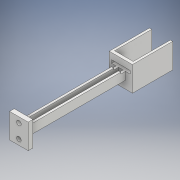
# Autodesk Inventor part: learnbotAgarreServo
Saved by Autodesk Inventor 2017 (Build 210142000, 142)
## iProperties
Part Number: learnbotAgarreServo
Material: Genérico
Document SubType Name: Modeling
Designer: rober
Density: 1 g/cm^3
Appearance: Valor por defecto
Author: rober
Autodesk Inventor part; units mm, degrees
ref_plane "YZ Plane" through (0, 0, 0) normal (1, 0, 0) x (0, 1, 0)
ref_plane "XZ Plane" through (0, 0, 0) normal (0, 1, 0) x (-1, 0, 0)
ref_plane "XY Plane" through (0, 0, 0) normal (0, 0, 1) x (1, 0, 0)
sketch "Boceto1" plane through (0, 0, 0) normal (0, 0, 1) x (1, 0, 0)
  line L0 (-0.3, 9.187) -> (-0.3, 6.787)
  line L1 (-0.3, 6.787) -> (0.9, 6.787)
  line L2 (0.9, 6.787) -> (0.9, 9.187)
  line L3 (0.9, 9.187) -> (1.05, 9.187)
  line L4 (1.05, 9.187) -> (1.05, 6.587)
  line L5 (0, 6.587) -> (-0.45, 6.587)
  line L6 (-0.45, 6.587) -> (-0.45, 9.187)
  line L7 (-0.45, 9.187) -> (-0.3, 9.187)
  line L8 (0.6, 0) -> (0.6, 6.587)
  line L9 (0.45, 6.587) -> (0.15, 6.587)
  line L10 (0, 6.587) -> (0, 0)
  line L11 (0, 0.3) -> (0.6, 0.3)
  line L12 (0.15, 0.3) -> (0.15, 6.587)
  line L13 (0.45, 0.3) -> (0.45, 6.587)
  line L14 (0.6, 6.587) -> (1.05, 6.587)
  line L15 (0, 0) -> (0.6, 0)
  point P0 (0, 0)
  constraints: 32 end point, 4 point on line
extrude "Extrusión1" add sketch "Boceto1" along normal blind 1.6 contours L0 L1 L2 L3 L4 L14 L8 L11 L13 L9 L12 L10 L5 L6 L7 | L11 L8 L15 L10
sketch "Boceto2" plane through (-0.3, 6.787, 0) normal (0, 1, 0) x (1, 0, 0)
  line L0 (1.2, 0) -> (0, 0) projected
  line L1 (0, 0) -> (0, -1.6) projected
  line L2 (1.2, -1.6) -> (0, -1.6) projected
  line L3 (1.2, 0) -> (1.2, -1.6) projected
  line L4 (0, -1.6) -> (0, -1.2)
  line L5 (0, -1.2) -> (0, -1)
  line L6 (0, -1) -> (1.2, -1)
  line L7 (1.2, 0) -> (1.2, -1.6) projected
  line L8 (0, -1.2) -> (1.2, -1.2)
  line L9 (1.2, -1.2) -> (1.2, -1)
  point P0 (0.3, 0)
  dimension "d2" = 0.4
  dimension "d3" = 0.2
  dimension "d4" = 1.2
  constraints: 10 end point, 4 point on line, 1 perpendicular
  measures "d2" distance of L1.end L4.end
  measures "d3" distance of L4.end L5.end
  measures "d4" distance of L4.end L8.end
extrude "Extrusión2" cut sketch "Boceto2" against normal blind 0.5 contours L3 L8 L1 L6
sketch "Boceto3" plane through (0.6, 0, 0) normal (1, 0, 0) x (0, 0, -1)
  line L0 (-1.6, 0.3) -> (0, 0.3) projected
  line L1 (-1, 6.587) -> (-1, 6.287) projected
  line L2 (-1, 6.287) -> (-1.2, 6.287) projected
  line L3 (-1.2, 6.287) -> (-1.2, 6.587) projected
  line L4 (-1.2, 6.587) -> (-1.6, 6.587) projected
  line L5 (-1.6, 0) -> (-1.6, 6.587) projected
  line L6 (0, 0) -> (-1.6, 0) projected
  line L7 (0, 0) -> (0, 6.587) projected
  line L8 (0, 6.587) -> (-1, 6.587) projected
  line L9 (-1.6, 0.3) -> (-1.6, 6.587) projected
  line L10 (-1.6, 0.3) -> (-1.2, 0.3)
  line L11 (-1.2, 0.3) -> (-1.2, 6.587)
  line L12 (-1.6, 6.587) -> (-1.2, 6.587)
  line L13 (-1.2, 6.587) -> (-1.2, 0.3)
  line L14 (-1.2, 0.3) -> (-1.6, 0.3)
  line L15 (-1.6, 0.3) -> (-1.6, 6.587)
  line L16 (0, 0.3) -> (0, 6.587) projected
  line L17 (0, 0.3) -> (-0.4, 0.3)
  line L18 (0, 0.3) -> (-1.6, 0.3) projected
  line L19 (0, 6.587) -> (-1.6, 6.587) projected
  line L20 (0, 6.587) -> (-0.4, 6.587)
  line L21 (-0.4, 6.587) -> (-0.4, 0.3)
  line L22 (-0.4, 0.3) -> (0, 0.3)
  line L23 (0, 0.3) -> (0, 6.587)
  point P0 (0, 0)
  dimension "d7" = 0.4
  dimension "d8" = 0.4
  constraints: 22 end point, 4 parallel, 2 horizontal, 2 perpendicular, 2 point on line
  measures "d7" distance of L0.start L10.end
  measures "d8" distance of L0.end L17.end
extrude "Extrusión3" cut sketch "Boceto3" against normal blind 0.9 contours L5 L4 L3 L11 L0 | L21 L8 L7 L0
sketch "Boceto4" plane through (0, 0.3, 0) normal (0, 1, 0) x (1, 0, 0)
  line L0 (0, 0) -> (0.6, 0) projected
  line L1 (0.6, 0) -> (0.6, -1.6) projected
  line L2 (0, -1.6) -> (0.6, -1.6) projected
  line L3 (0, 0) -> (0, -1.6) projected
  line L4 (0, -1.6) -> (0.6, -1.6) projected
  circle A0 centre (0.3, -1.35) radius 0.15
  line L5 (0, 0) -> (0, -1.6) projected
  circle A1 centre (0.3, -0.25) radius 0.15
  dimension "d12" = 0.3
  constraints: 2 centre point
  measures "d12" diameter of A0
extrude "Extrusión4" cut sketch "Boceto4" against normal blind 10 contours A0 | A1
sketch "Boceto5" plane through (0.6, 0, 0) normal (1, 0, 0) x (0, 0, -1)
  line L0 (-1.2, 0.3) -> (-1.6, 0.3) projected
  line L1 (-1.6, 0) -> (-1.6, 0.3) projected
  line L2 (0, 0) -> (-1.6, 0) projected
  line L3 (0, 0) -> (0, 0.3) projected
  line L4 (0, 0.3) -> (-0.4, 0.3) projected
  line L5 (-0.4, 0.3) -> (-0.4, 6.587) projected
  line L6 (-0.4, 6.587) -> (-1, 6.587) projected
  line L7 (-1, 6.587) -> (-1, 6.287) projected
  line L8 (-1, 6.287) -> (-1.2, 6.287) projected
  line L9 (-1.2, 6.287) -> (-1.2, 0.3) projected
  line L10 (-1.2, 6.287) -> (-1.2, 0.3) projected
  line L11 (-1.2, 6.287) -> (-1.1, 6.287)
  line L12 (-1, 6.287) -> (-1.2, 6.287) projected
  line L13 (-1.2, 0.3) -> (-1.1, 0.3)
  line L14 (-1.1, 0.3) -> (-1.1, 6.287)
  line L15 (-0.4, 0.3) -> (-0.5, 0.3)
  line L16 (-0.4, 0.3) -> (-1.2, 0.3) projected
  line L17 (-0.5, 0.3) -> (-0.5, 6.587)
  line L18 (-0.4, 0.3) -> (-0.4, 6.587) projected
  line L19 (-0.4, 6.587) -> (-0.4, 0.3)
  line L20 (-1.2, 0.3) -> (-1.2, 6.287)
  point P0 (0, 0)
  dimension "d15" = 0.1
  dimension "d16" = 0.1
  dimension "d17" = 0.1
  constraints: 14 end point, 2 parallel, 2 point on line, 1 horizontal, 1 midpoint, 1 vertical
  measures "d15" distance of L8.end L11.end
  measures "d16" distance of L0.start L13.end
  measures "d17" distance of L4.end L15.end
extrude "Extrusión5" cut sketch "Boceto5" against normal blind 10 contours L9 L8 L14 L13 | L17 L6 L5 L15
sketch "Boceto6" plane through (0, 0, 0) normal (0, -1, 0) x (1, 0, 0)
  line L0 (0.9, 1.6) -> (0.9, 0)
  line L1 (0.9, 0) -> (-0.3, 0)
  line L2 (-0.3, 0) -> (-0.3, 1.6)
  line L3 (-0.3, 1.6) -> (0.9, 1.6)
  circle A0 centre (0.3, 1.25) radius 0.15
  circle A1 centre (0.3, 0.35) radius 0.15
  line L4 (0, 1.6) -> (0.6, 1.6) projected
  line L5 (0, 0) -> (0.6, 0) projected
  constraints: 8 end point, 2 centre point
extrude "Extrusión6" add sketch "Boceto6" against normal blind 0.3 contours L0 L1 L2 L3 | A0 | A1
sketch "Boceto7" plane through (0.9, 0, 0) normal (0, -1, 0) x (1, 0, 0)
  line L0 (0, 1.6) -> (0, 0)
  line L1 (0, 0) -> (-1.2, 0)
  line L2 (-1.2, 0) -> (-1.2, 1.6)
  line L3 (-1.2, 1.6) -> (0, 1.6)
  circle A0 centre (-0.6, 1.25) radius 0.15
  circle A1 centre (-0.6, 0.35) radius 0.15
  line L4 (-0.9, 1.6) -> (-0.3, 1.6)
  line L5 (-0.9, 0) -> (-0.3, 0)
  line L6 (-1.2, 0) -> (-1.2, 1.6) projected
  point P0 (-0.9, 0)
  constraints: 12 end point, 2 centre point
extrude "Extrusión7" cut sketch "Boceto7" against normal blind 0.5 contours A0 | A1
